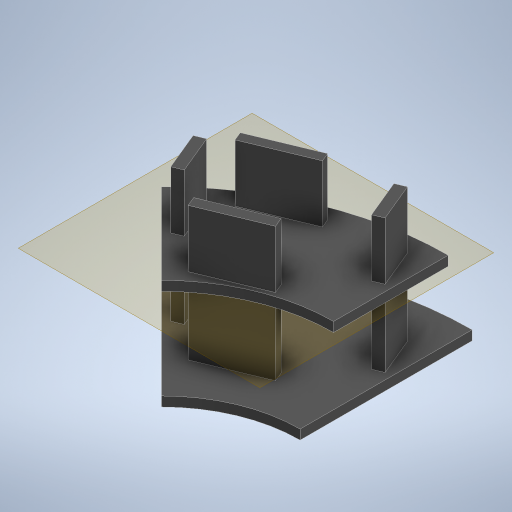
# Autodesk Inventor part: Carousel Container Plate
Saved by Autodesk Inventor 2023 (Build 270158000, 158)
## iProperties
Created: 2022-11-11
Part Number: Carousel Container Plate
Material: PLA Plastic
Document SubType Name: Modeling
Designer: cheng
Density: 0.373679 g/cm^3
Appearance: Generic
Mass: 259.485 g
Surface Area: 1676.4 cm^2
Volume: 694.407 cm^3
Author: cheng
Autodesk Inventor part; units mm, degrees
ref_plane "YZ Plane" through (0, 0, 0) normal (1, 0, 0) x (0, 1, 0)
ref_plane "XZ Plane" through (0, 0, 0) normal (0, 1, 0) x (-1, 0, 0)
ref_plane "XY Plane" through (0, 0, 0) normal (0, 0, 1) x (1, 0, 0)
sketch "Sketch1" plane through (0, 0, 0) normal (0, 1, 0) x (-1, 0, 0)
  circle A0 centre (0, 0) radius 145
  circle A1 centre (0, 0) radius 325
  line L0 (0, 0) -> (325, 0)
  line L1 (0, 0) -> (0, -325)
  line L2 (0, 0) -> (229.8097, -229.8097)
  line L3 (229.8097, -229.8097) -> (0, -145) construction
  line L4 (9.0406, -217.8104) -> (147.6225, -160.4079)
  line L5 (147.6225, -160.4079) -> (178.2372, -234.3183)
  line L6 (178.2372, -234.3183) -> (39.6553, -291.7208)
  line L7 (39.6553, -291.7208) -> (9.0406, -217.8104)
  line L8 (102.5305, -102.5305) -> (-3.7965, -324.9778) construction
  circle A2 centre (0, 0) radius 306.4883 construction
  line L9 (178.2372, -234.3183) -> (9.0406, -217.8104) construction
  line L10 (147.6225, -160.4079) -> (39.6553, -291.7208) construction
  line L11 (93.6389, -226.0643) -> (108.9463, -263.0195) construction
  line L12 (0, 0) -> (124.3721, -300.2608) construction
  line L13 (217.8104, -9.0406) -> (291.7208, -39.6553)
  line L14 (160.4079, -147.6225) -> (217.8104, -9.0406)
  line L15 (234.3183, -178.2372) -> (160.4079, -147.6225)
  line L16 (291.7208, -39.6553) -> (234.3183, -178.2372)
  line L17 (160.4079, 147.6225) -> (234.3183, 178.2372)
  line L18 (217.8104, 9.0406) -> (160.4079, 147.6225)
  line L19 (291.7208, 39.6553) -> (217.8104, 9.0406)
  line L20 (234.3183, 178.2372) -> (291.7208, 39.6553)
  line L21 (9.0406, 217.8104) -> (39.6553, 291.7208)
  line L22 (147.6225, 160.4079) -> (9.0406, 217.8104)
  line L23 (178.2372, 234.3183) -> (147.6225, 160.4079)
  line L24 (39.6553, 291.7208) -> (178.2372, 234.3183)
  line L25 (-147.6225, 160.4079) -> (-178.2372, 234.3183)
  line L26 (-9.0406, 217.8104) -> (-147.6225, 160.4079)
  line L27 (-39.6553, 291.7208) -> (-9.0406, 217.8104)
  line L28 (-178.2372, 234.3183) -> (-39.6553, 291.7208)
  line L29 (-217.8104, 9.0406) -> (-291.7208, 39.6553)
  line L30 (-160.4079, 147.6225) -> (-217.8104, 9.0406)
  line L31 (-234.3183, 178.2372) -> (-160.4079, 147.6225)
  line L32 (-291.7208, 39.6553) -> (-234.3183, 178.2372)
  line L33 (-160.4079, -147.6225) -> (-234.3183, -178.2372)
  line L34 (-217.8104, -9.0406) -> (-160.4079, -147.6225)
  line L35 (-291.7208, -39.6553) -> (-217.8104, -9.0406)
  line L36 (-234.3183, -178.2372) -> (-291.7208, -39.6553)
  line L37 (-9.0406, -217.8104) -> (-39.6553, -291.7208)
  line L38 (-147.6225, -160.4079) -> (-9.0406, -217.8104)
  line L39 (-178.2372, -234.3183) -> (-147.6225, -160.4079)
  line L40 (-39.6553, -291.7208) -> (-178.2372, -234.3183)
  circle A3 centre (0, 0) radius 235 construction
  point P0 (263.0195, -108.9463)
  point P1 (263.0195, 108.9463)
  point P2 (108.9463, 263.0195)
  point P3 (-108.9463, 263.0195)
  point P4 (-263.0195, 108.9463)
  point P5 (-263.0195, -108.9463)
  point P6 (-108.9463, -263.0195)
  dimension "d1" = 180
  dimension "d3" = 45
  dimension "d4" = 650
  dimension "d11" = 150
  dimension "d12" = 80
  dimension "d13" = 22.5
  dimension "d16" = 360
  dimension "d18" = 90
  constraints: 82 end point, 7 point on circle, 4 centre point, 4 coincident, 2 midpoint, 2 parallel, 2 perpendicular, 2 point on line, 1 collinear, 1 horizontal, 73 other
  measures "d1" radial gap between concentric circles of A0 A1
  measures "d3" angle of L1 L2
  measures "d4" diameter of A1
  measures "d11" distance of L5.end L6.end
  measures "d12" distance of L6.end L4.start
  measures "d13" angle of L2 L12
  measures "d18" radial gap between concentric circles of A1 A3
extrude "Extrusion1" add sketch "Sketch1" along normal blind 10 contours A0 L2 A1 L1 | L4 L5 L6 L7
sketch "Sketch2" plane through (0, 10, 0) normal (0, 1, 0) x (1, 0, 0)
  circle A0 centre (0, 0) radius 325
  circle A1 centre (0, 0) radius 145
  line L0 (0, 0) -> (-325, 0)
  line L1 (0, 145) -> (0, 325) projected
  line L2 (0, 0) -> (0, 325)
  arc A2 (0, 325) -> (-229.8097, 229.8097) centre (0, 0) ccw projected
  line L3 (0, 0) -> (-229.8097, 229.8097)
  circle A3 centre (0, 0) radius 235 construction
  line L4 (0, 0) -> (-124.3721, 300.2608) construction
  line L5 (-5.3323, 208.8578) -> (-143.9142, 151.4553)
  line L6 (-143.9142, 151.4553) -> (-174.5289, 225.3656)
  line L7 (-174.5289, 225.3656) -> (-35.947, 282.7681)
  line L8 (-35.947, 282.7681) -> (-5.3323, 208.8578)
  line L9 (-5.3323, 208.8578) -> (-174.5289, 225.3656) construction
  line L10 (-143.9142, 151.4553) -> (-35.947, 282.7681) construction
  circle A4 centre (0, 0) radius 195
  line L11 (-208.8578, 5.3323) -> (-282.7681, 35.947)
  line L12 (-151.4553, 143.9142) -> (-208.8578, 5.3323)
  line L13 (-225.3656, 174.5289) -> (-151.4553, 143.9142)
  line L14 (-282.7681, 35.947) -> (-225.3656, 174.5289)
  line L15 (-208.8578, 5.3323) -> (-225.3656, 174.5289) construction
  line L16 (-151.4553, 143.9142) -> (-282.7681, 35.947) construction
  line L17 (-151.4553, -143.9142) -> (-225.3656, -174.5289)
  line L18 (-208.8578, -5.3323) -> (-151.4553, -143.9142)
  line L19 (-282.7681, -35.947) -> (-208.8578, -5.3323)
  line L20 (-225.3656, -174.5289) -> (-282.7681, -35.947)
  line L21 (-151.4553, -143.9142) -> (-282.7681, -35.947) construction
  line L22 (-208.8578, -5.3323) -> (-225.3656, -174.5289) construction
  line L23 (-5.3323, -208.8578) -> (-35.947, -282.7681)
  line L24 (-143.9142, -151.4553) -> (-5.3323, -208.8578)
  line L25 (-174.5289, -225.3656) -> (-143.9142, -151.4553)
  line L26 (-35.947, -282.7681) -> (-174.5289, -225.3656)
  line L27 (-5.3323, -208.8578) -> (-174.5289, -225.3656) construction
  line L28 (-143.9142, -151.4553) -> (-35.947, -282.7681) construction
  line L29 (143.9142, -151.4553) -> (174.5289, -225.3656)
  line L30 (5.3323, -208.8578) -> (143.9142, -151.4553)
  line L31 (35.947, -282.7681) -> (5.3323, -208.8578)
  line L32 (174.5289, -225.3656) -> (35.947, -282.7681)
  line L33 (143.9142, -151.4553) -> (35.947, -282.7681) construction
  line L34 (5.3323, -208.8578) -> (174.5289, -225.3656) construction
  line L35 (208.8578, -5.3323) -> (282.7681, -35.947)
  line L36 (151.4553, -143.9142) -> (208.8578, -5.3323)
  line L37 (225.3656, -174.5289) -> (151.4553, -143.9142)
  line L38 (282.7681, -35.947) -> (225.3656, -174.5289)
  line L39 (208.8578, -5.3323) -> (225.3656, -174.5289) construction
  line L40 (151.4553, -143.9142) -> (282.7681, -35.947) construction
  line L41 (151.4553, 143.9142) -> (225.3656, 174.5289)
  line L42 (208.8578, 5.3323) -> (151.4553, 143.9142)
  line L43 (282.7681, 35.947) -> (208.8578, 5.3323)
  line L44 (225.3656, 174.5289) -> (282.7681, 35.947)
  line L45 (151.4553, 143.9142) -> (282.7681, 35.947) construction
  line L46 (208.8578, 5.3323) -> (225.3656, 174.5289) construction
  line L47 (5.3323, 208.8578) -> (35.947, 282.7681)
  line L48 (143.9142, 151.4553) -> (5.3323, 208.8578)
  line L49 (174.5289, 225.3656) -> (143.9142, 151.4553)
  line L50 (35.947, 282.7681) -> (174.5289, 225.3656)
  line L51 (5.3323, 208.8578) -> (174.5289, 225.3656) construction
  line L52 (143.9142, 151.4553) -> (35.947, 282.7681) construction
  line L53 (-155.3947, 179.1716) -> (-165.3947, 175.0295)
  line L54 (-165.3947, 175.0295) -> (-181.9633, 215.0295)
  line L55 (-181.9633, 215.0295) -> (-171.9633, 219.1716)
  line L56 (-171.9633, 219.1716) -> (-155.3947, 179.1716)
  line L57 (-155.3947, 179.1716) -> (-181.9633, 215.0295) construction
  line L58 (-165.3947, 175.0295) -> (-171.9633, 219.1716) construction
  line L59 (-16.8128, 236.5742) -> (-6.8128, 240.7163)
  line L60 (-6.8128, 240.7163) -> (-23.3813, 280.7163)
  line L61 (-23.3813, 280.7163) -> (-33.3813, 276.5742)
  line L62 (-16.8128, 236.5742) -> (-23.3813, 280.7163) construction
  line L63 (-6.8128, 240.7163) -> (-33.3813, 276.5742) construction
  line L64 (-60.7651, 185.8968) -> (-125.4366, 159.1089)
  line L65 (-125.4366, 159.1089) -> (-121.2945, 149.1089)
  line L66 (-121.2945, 149.1089) -> (-56.6229, 175.8968)
  line L67 (-56.6229, 175.8968) -> (-60.7651, 185.8968)
  line L68 (-60.7651, 185.8968) -> (-121.2945, 149.1089) construction
  line L69 (-125.4366, 159.1089) -> (-56.6229, 175.8968) construction
  line L70 (-91.3798, 259.8071) -> (-156.0513, 233.0193)
  line L71 (-156.0513, 233.0193) -> (-159.8782, 242.2581)
  line L72 (-159.8782, 242.2581) -> (-95.2066, 269.0459)
  line L73 (-95.2066, 269.0459) -> (-91.3798, 259.8071)
  point P0 (-89.9306, 217.1117)
  point P1 (-217.1117, 89.9306)
  point P2 (-217.1117, -89.9306)
  point P3 (-89.9306, -217.1117)
  point P4 (89.9306, -217.1117)
  point P5 (217.1117, -89.9306)
  point P6 (217.1117, 89.9306)
  point P7 (89.9306, 217.1117)
  point P8 (-68.8241, 166.1562)
  point P9 (-33.3813, 276.5742)
  point P10 (-16.8128, 236.5742)
  point P11 (-155.3947, 179.1716)
  point P12 (-60.7651, 185.8968)
  point P13 (-125.4366, 159.1089)
  point P14 (-156.0513, 233.0193)
  point P15 (-91.3798, 259.8071)
  dimension "d22" = 180
  dimension "d23" = 650
  dimension "d24" = 90
  dimension "d25" = 80
  dimension "d26" = 150
  dimension "d27" = 50
  dimension "d30" = 360
  dimension "d32" = 40
  dimension "d33" = 10
  dimension "d34" = 10
  dimension "d39" = 30
  dimension "d40" = 20
  dimension "d46" = 10
  dimension "d47" = 70
  dimension "d48" = 20
  dimension "d49" = 70
  constraints: 146 end point, 8 parallel, 4 coincident, 4 collinear, 4 perpendicular, 4 symmetric about line, 3 centre point, 2 midpoint, 2 point on circle, 1 horizontal, 1 point on line, 1 tangent, 1 vertical alignment, 90 other
  measures "d23" diameter of A0
  measures "d24" radial gap between concentric circles of A0 A3
  measures "d25" distance of L7.end L5.start
  measures "d26" distance of L5.start L5.end
  measures "d32" vertical distance of L53.end L54.end
  measures "d33" horizontal distance of L54.end L55.end
  measures "d34" vertical distance of L64.end L65.end
  measures "d39" distance between parallel lines of L5 L53
  measures "d40" distance between parallel lines of L6 L65
  measures "d46" distance between parallel lines of L72 L70
  measures "d47" distance between parallel lines of L73 L71
  measures "d48" distance between parallel lines of L6 L71
  measures "d49" distance between parallel lines of L67 L65
extrude "Extrusion2" add sketch "Sketch2" along normal blind 140 contours L67 L66 L65 A4 | A4 L5 L67 | L65 L5 A4 | L8 L61 L60 L59 | L53 L54 L55 L6 | L7 L71 L72 L73
ref_plane "Work Plane1" through (0, 80, 0) normal (0, 1, 0) x (1, 0, 0)
sketch "Sketch4" plane through (0, 80, 0) normal (0, 1, 0) x (1, 0, 0)
  line L0 (-23.3813, 280.7163) -> (-6.8128, 240.7163) projected
  line L1 (-6.8128, 240.7163) -> (-16.8128, 236.5742) projected
  line L2 (-16.8128, 236.5742) -> (-33.3813, 276.5742) projected
  line L3 (-33.3813, 276.5742) -> (-23.3813, 280.7163) projected
  line L4 (-165.3947, 175.0295) -> (-181.9633, 215.0295) projected
  line L5 (-181.9633, 215.0295) -> (-171.9633, 219.1716) projected
  line L6 (-171.9633, 219.1716) -> (-155.3947, 179.1716) projected
  line L7 (-155.3947, 179.1716) -> (-165.3947, 175.0295) projected
  line L8 (-56.6229, 175.8968) -> (-121.2945, 149.1089) projected
  line L9 (-121.2945, 149.1089) -> (-125.4366, 159.1089) projected
  line L10 (-125.4366, 159.1089) -> (-60.7651, 185.8968) projected
  line L11 (-60.7651, 185.8968) -> (-56.6229, 175.8968) projected
  arc A0 (0, 145) -> (-102.5305, 102.5305) centre (0, 0) ccw projected
  line L12 (0, 145) -> (0, 325) projected
  arc A1 (0, 325) -> (-229.8097, 229.8097) centre (0, 0) ccw projected
  line L13 (-229.8097, 229.8097) -> (-102.5305, 102.5305) projected
  arc A2 (0, 180) -> (-127.2792, 127.2792) centre (0, 0) ccw
  arc A3 (0, 300) -> (-212.132, 212.132) centre (0, 0) ccw
  dimension "d44" = 35
  dimension "d50" = 25
  constraints: 4 point on circle, 4 point on line, 2 centre point, 2 coincident
  measures "d44" radial gap between concentric circles of A0 A2
  measures "d50" radial gap between concentric circles of A1 A3
extrude "Extrusion3" add sketch "Sketch4" along normal blind 10 contours A2 L13 A3 L12
body "Solid1"
